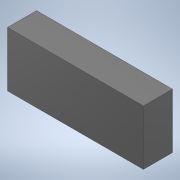
# Autodesk Inventor part: usbHub
Saved by Autodesk Inventor 2021.2 (Build 252289000, 289)
## iProperties
Created: 2021-02-17
Part Number: usbHub
Material: PC/ABS Plastic
Document SubType Name: Modeling
Designer: robst
Density: 0.357273 g/cm^3
Appearance: Smooth - Black
Author: robst
Autodesk Inventor part; units mm, degrees
ref_plane "YZ Plane" through (0, 0, 0) normal (1, 0, 0) x (0, 1, 0)
ref_plane "XZ Plane" through (0, 0, 0) normal (0, 1, 0) x (-1, 0, 0)
ref_plane "XY Plane" through (0, 0, 0) normal (0, 0, 1) x (1, 0, 0)
sketch "Sketch1" plane through (0, 0, 0) normal (0, 0, 1) x (1, 0, 0)
  line L0 (-54.61, -22.098) -> (54.61, -22.098)
  line L1 (54.61, -22.098) -> (54.61, 22.098)
  line L2 (54.61, 22.098) -> (-54.61, 22.098)
  line L3 (-54.61, 22.098) -> (-54.61, -22.098)
  line L4 (-54.61, -22.098) -> (54.61, 22.098) construction
  line L5 (54.61, -22.098) -> (-54.61, 22.098) construction
  point P0 (0, 0)
  dimension "d0" = 109.22
  dimension "d1" = 44.196
  constraints: 12 end point, 2 midpoint, 2 parallel, 1 horizontal, 1 perpendicular
  measures "d0" distance of L1.end L2.end
  measures "d1" distance of L2.end L0.start
extrude "Extrusion1" add sketch "Sketch1" along normal blind 23.368
body "Solid1"
